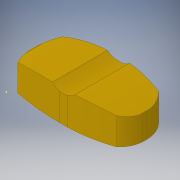
# Autodesk Inventor part: SSOK
Saved by Autodesk Inventor 2019 (Build 230136000, 136)
## iProperties
Created: 2020-02-15
Part Number: SSOK
Material: Generic
Document SubType Name: Modeling
Designer: brosemej
Density: 1 g/cm^3
Appearance: Gold
Author: brosemej
Autodesk Inventor part; units mm, degrees
ref_plane "YZ Plane" through (0, 0, 0) normal (1, 0, 0) x (0, 1, 0)
ref_plane "XZ Plane" through (0, 0, 0) normal (0, 1, 0) x (-1, 0, 0)
ref_plane "XY Plane" through (0, 0, 0) normal (0, 0, 1) x (1, 0, 0)
sketch "Sketch1" plane through (0, 0, 0) normal (0, 1, 0) x (-1, 0, 0)
  line L0 (-3, 0) -> (-97, 0)
  line L1 (-100, -3) -> (-100, -47)
  line L2 (-97, -50) -> (-3, -50)
  line L3 (0, -47) -> (0, -3)
  line L4 (0, -50) -> (0, -25)
  line L5 (0, -25) -> (-12.1, -25)
  circle A0 centre (-12.1, -25) radius 2.4
  line L6 (-12.1, -25) -> (-87.8936, -25)
  circle A1 centre (-87.8936, -25) radius 2.4
  arc A2 (0, -3) -> (-3, 0) centre (-3, -3) ccw
  arc A3 (-3, -50) -> (0, -47) centre (-3, -47) ccw
  arc A4 (-97, 0) -> (-100, -3) centre (-97, -3) ccw
  arc A5 (-100, -47) -> (-97, -50) centre (-97, -47) ccw
  point P0 (0, 0)
  point P1 (-100, -50)
  point P2 (-100, 0)
  dimension "d0" = 100
  dimension "d1" = 50
  dimension "d2" = 25
  dimension "d3" = 12.1
  dimension "d4" = 4.8
  dimension "d5" = 75.7936
  dimension "d6" = 4.8
  dimension "d7" = 3
  constraints: 14 end point, 8 point on circle, 8 point on line, 8 tangent, 6 centre point, 3 equal radius, 2 coincident, 2 horizontal, 2 parallel, 2 perpendicular, 1 midpoint
  measures "d0" distance of L4.start point (-100, -50)
  measures "d1" distance of point (-100, -50) point (-100, 0)
  measures "d2" distance of L4.start L4.end
  measures "d3" distance of L4.end L5.end
  measures "d4" diameter of A0
  measures "d5" distance of L6.start L6.end
  measures "d6" diameter of A1
  measures "d7" radius of A2
extrude "Extrusion1" add sketch "Sketch1" along normal blind 10
sketch "Sketch2" plane through (0, 10, 0) normal (0, 1, 0) x (1, 0, 0)
  line L0 (2, 0) -> (98, 0)
  line L1 (100, 2) -> (100, 48)
  line L2 (98, 50) -> (2, 50)
  line L3 (0, 48) -> (0, 2)
  arc A0 (98, 0) -> (100, 2) centre (98, 2) ccw
  arc A1 (0, 2) -> (2, 0) centre (2, 2) ccw
  arc A2 (2, 50) -> (0, 48) centre (2, 48) ccw
  arc A3 (100, 48) -> (98, 50) centre (98, 48) ccw
  point P0 (0, 0)
  dimension "d10" = 2
  constraints: 8 end point, 8 point on circle, 8 tangent, 4 centre point, 3 equal radius, 2 parallel, 2 point on line, 1 horizontal, 1 perpendicular
  measures "d10" radius of A0
extrude "Extrusion2" add sketch "Sketch2" along normal blind 18.3
sketch "Sketch3" plane through (3, 0, 0) normal (0, 0, 1) x (1, 0, 0)
  point P0 (-3, 0)
sketch "Sketch4" plane through (0, 28.3, 0) normal (0, 1, 0) x (1, 0, 0)
  line L0 (3, 0) -> (97, 0) projected
  arc A0 (6.1709, 4.1832) -> (50, 0) centre (48.8144, 219.278) ccw
  line L1 (0, 47) -> (0, 3) projected
  arc A1 (0, 25) -> (6.1709, 4.1832) centre (35.6265, 24.238) ccw
  arc A2 (6.1709, 44.2928) -> (0, 25) centre (35.6265, 24.238) ccw
  line L2 (97, 50) -> (3, 50) projected
  arc A3 (50, 50) -> (6.1709, 44.2928) centre (53.6635, -149.2845) ccw
  arc A4 (92.3505, 44.2928) -> (50, 50) centre (45.5073, -143.3251) ccw
  line L3 (100, 3) -> (100, 47) projected
  arc A5 (100, 25) -> (92.3505, 44.2928) centre (73.1068, 25.5) ccw
  arc A6 (92.3505, 6.7071) -> (100, 25) centre (77.2233, 23.7786) ccw
  arc A7 (50, 0) -> (92.3505, 6.7071) centre (52.254, 122.8285) ccw
  point P0 (0, 0)
  constraints: 18 point on circle, 8 centre point, 4 midpoint, 1 concentric
extrude "Extrusion3" cut sketch "Sketch4" against normal blind 28.1 keep common part
sketch "Sketch5" plane through (47.6287, 28.3, 0) normal (0, 0, 1) x (1, 0, 0)
  line L0 (0, 0) -> (6.8792, 0) projected
  line L1 (3.4396, 0) -> (-6.5604, 0)
  line L2 (3.4396, 0) -> (13.4396, 0)
  line L3 (6.8792, 0) -> (44.7218, 0) projected
  arc A0 (-6.5604, 0) -> (13.4396, 0) centre (3.4396, 11.1803) ccw
  point P0 (-47.6287, -28.3)
  dimension "d15" = 10
  dimension "d16" = 10
  dimension "d17" = 15
  constraints: 4 end point, 2 point on circle, 1 centre point, 1 collinear, 1 midpoint, 1 point on line
  measures "d15" distance of L1.start L1.end
  measures "d16" distance of L1.start L2.end
  measures "d17" radius of A0
extrude "Extrusion4" cut sketch "Sketch5" against normal blind 50
sketch "Sketch6" plane through (47.6287, 0.2, 0) normal (0, 0, 1) x (1, 0, 0)
  arc A0 (-6.5604, 28.1) -> (-46.762, 22.2881) centre (-6.5604, -113.8444) ccw
  arc A1 (52.1024, 22.2904) -> (13.4396, 28.1) centre (13.4396, -103.4557) ccw
  line L0 (52.1024, 22.2904) -> (52.3713, 28.1)
  line L1 (52.3713, 28.1) -> (13.4396, 28.1)
  line L2 (-6.5604, 28.1) -> (-47.6287, 28.1)
  line L3 (-47.6287, 28.1) -> (-46.762, 22.2881)
  point P0 (-47.6287, -0.2)
  constraints: 8 end point, 5 point on circle, 2 centre point, 2 horizontal, 2 tangent
extrude "Extrusion5" cut sketch "Sketch6" against normal blind 50
sketch "Sketch7" plane through (47.6287, 0.2, 0) normal (0, 0, 1) x (1, 0, 0)
  line L0 (-47.6287, 28.1) -> (-47.6287, 0) projected
  arc A0 (-46.762, 22.2881) -> (-47.6287, 21.9584) centre (-45.4512, 17.5372) ccw
  line L1 (-47.6287, 21.9584) -> (-47.6287, 28.1)
  line L2 (-46.762, 22.2881) -> (-47.6287, 28.1)
  point P0 (-47.6287, -0.2)
  constraints: 4 end point, 2 point on circle, 1 centre point, 1 collinear, 1 point on line
extrude "Extrusion6" cut sketch "Sketch7" against normal blind 50
sketch "Sketch8" plane through (47.6287, 0.2, 0) normal (0, 0, 1) x (1, 0, 0)
  line L0 (52.3713, 28.1) -> (52.3713, 0) projected
  line L1 (52.1024, 22.2904) -> (52.3713, 28.1) projected
  arc A0 (52.3713, 22.1965) -> (52.1024, 22.2904) centre (49.9324, 15.6487) ccw
  line L2 (52.1024, 22.2904) -> (52.3713, 28.1)
  line L3 (52.3713, 28.1) -> (52.3713, 22.1965)
  point P0 (-47.6287, -0.2)
  constraints: 4 end point, 2 point on circle, 1 centre point, 1 point on line, 1 vertical
extrude "Extrusion7" cut sketch "Sketch8" against normal blind 50
body "Solid1"
